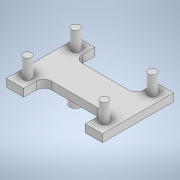
# Autodesk Inventor part: IMU mount
Saved by Autodesk Inventor 2022.6 (Build 266554000, 554)
## iProperties
Created: 2024-11-16
Part Number: IMU mount
Material: Generic
Document SubType Name: Modeling
Designer: Zhong
Density: 1 g/cm^3
Appearance: Default
Author: Zhong
Autodesk Inventor part; units mm, degrees
ref_plane "YZ Plane" through (0, 0, 0) normal (1, 0, 0) x (0, 1, 0)
ref_plane "XZ Plane" through (0, 0, 0) normal (0, 1, 0) x (-1, 0, 0)
ref_plane "XY Plane" through (0, 0, 0) normal (0, 0, 1) x (1, 0, 0)
sketch "Sketch1" plane through (0, 0, 0) normal (0, 1, 0) x (-1, 0, 0)
  line L0 (12.5, 9.25) -> (-12.5, 9.25)
  line L1 (-12.5, 9.25) -> (-12.5, -9.25)
  line L2 (-12.5, -9.25) -> (12.5, -9.25)
  line L3 (12.5, -9.25) -> (12.5, 9.25)
  line L4 (12.5, 9.25) -> (-12.5, -9.25) construction
  line L5 (-12.5, 9.25) -> (12.5, -9.25) construction
  line L6 (8, -4) -> (-8, -4)
  line L7 (-8, 4) -> (8, 4)
  line L8 (-17.5, 0) -> (17.5, 0) projected
  line L9 (8, -4) -> (8, -9.25)
  line L10 (8, 4) -> (8, 9.25)
  line L11 (-8, -4) -> (-8, -9.25)
  line L12 (-8, 4) -> (-8, 9.25)
  line L13 (0, -12.95) -> (0, 12.95) projected
  point P0 (0, 0)
  dimension "d0" = 25
  dimension "d1" = 18.5
  dimension "d24" = 8
  dimension "d25" = 16
  constraints: 24 end point, 6 point on line, 3 horizontal, 2 collinear, 2 midpoint, 2 parallel, 2 perpendicular, 1 vertical, 2 other
  measures "d0" distance of L0.start L0.end
  measures "d1" distance of L1.end L0.end
  measures "d24" distance between parallel lines of L7 L6
  measures "d25" distance between parallel lines of L11 L9
extrude "Extrusion1" add sketch "Sketch1" along normal blind 2 contours L3 L8 L13 L7 L10 L0 | L3 L2 L9 L6 L13 L8 | L13 L6 L11 L2 L1 L8 | L8 L1 L0 L12 L7 L13
sketch "Sketch2" plane through (0, 2, 0) normal (0, 1, 0) x (1, 0, 0)
  line L0 (17.5, 0) -> (-17.5, 0) projected
  line L1 (0, 12.95) -> (0, -12.95) projected
  line L2 (-10, -6.25) -> (10, -6.25) construction
  line L3 (10, -6.25) -> (10, 6.25) construction
  line L4 (10, 6.25) -> (-10, 6.25) construction
  line L5 (-10, 6.25) -> (-10, -6.25) construction
  line L6 (-10, -6.25) -> (10, 6.25) construction
  line L7 (10, -6.25) -> (-10, 6.25) construction
  line L8 (-10, 0) -> (10, 0) construction
  circle A0 centre (10, -6.25) radius 1.05
  circle A1 centre (10, 6.25) radius 1.05
  circle A2 centre (-10, 6.25) radius 1.05
  circle A3 centre (-10, -6.25) radius 1.05
  point P0 (0, 0)
  dimension "d5" = 20
  dimension "d6" = 12.5
  dimension "d10" = 2.1
  constraints: 14 end point, 6 midpoint, 4 centre point, 4 coincident, 3 equal radius, 2 parallel, 1 collinear, 1 perpendicular
  measures "d5" distance of L2.start L2.end
  measures "d6" distance of L3.end L2.end
  measures "d10" diameter of A3
extrude "Extrusion2" add sketch "Sketch2" along normal blind 5
sketch "Sketch5" plane through (0, 0, 0) normal (0, -1, 0) x (1, 0, 0)
  line L0 (0, 12.95) -> (0, -12.95) projected
  line L1 (-17.5, 0) -> (17.5, 0) projected
  circle A0 centre (-4.75, -1) radius 1.5
  circle A1 centre (4.75, -1) radius 1.5
  point P0 (0, 0)
  dimension "d26" = 3
  dimension "d27" = 3
  dimension "d28" = 1
  dimension "d29" = 9.5
  constraints: 2 centre point, 1 horizontal alignment, 1 symmetric about line
  measures "d26" diameter of A0
  measures "d27" diameter of A1
  measures "d28" distance from line of L1 A0.centre
  measures "d29" distance of A1.centre A0.centre
extrude "Extrusion4" add sketch "Sketch5" along normal blind 5
fillet "Fillet1" radius 2 4 edges at (-8, 1, 4) (8, 1, 4) (8, 1, -4) (-8, 1, -4)
body "Solid1"
